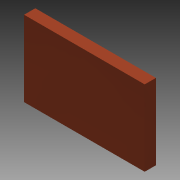
# Autodesk Inventor part: Heatsink cu base
Saved by Autodesk Inventor 2015 (Build 190159000, 159)
## iProperties
Created: 2015-08-21
Part Number: Heatsink cu base
Material: Copper
Document SubType Name: Modeling
Designer: Kyle
Density: 8.94 g/cm^3
Appearance: Copper - Satin
Author: Kyle
Autodesk Inventor part; units mm, degrees
ref_plane "YZ Plane" through (0, 0, 0) normal (1, 0, 0) x (0, 1, 0)
ref_plane "XZ Plane" through (0, 0, 0) normal (0, 1, 0) x (-1, 0, 0)
ref_plane "XY Plane" through (0, 0, 0) normal (0, 0, 1) x (1, 0, 0)
sketch "Sketch1" plane through (0, 0, 0) normal (0, 0, 1) x (1, 0, 0)
  line L0 (0, 0) -> (74.93, 0)
  line L1 (74.93, 0) -> (74.93, -46.99)
  line L2 (74.93, -46.99) -> (0, -46.99)
  line L3 (0, -46.99) -> (0, 0)
  dimension "d0" = 74.93
  dimension "d1" = 46.99
  constraints: 8 end point, 2 parallel, 1 horizontal, 1 perpendicular
  measures "d0" distance of L0.start L0.end
  measures "d1" distance of L2.end L0.start
extrude "Extrusion1" add sketch "Sketch1" along normal blind 6.985
body "Solid1"
